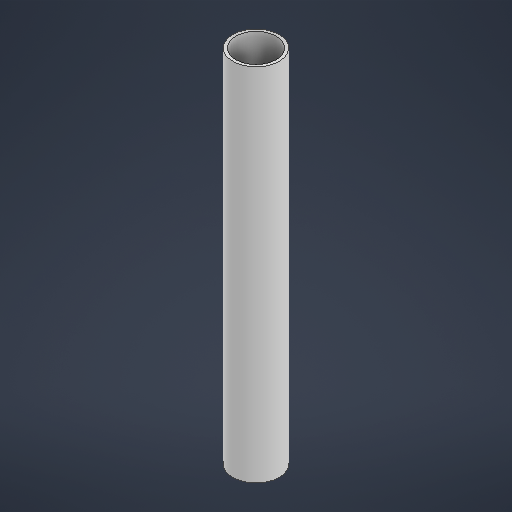
# Autodesk Inventor part: Fuel Tank
Saved by Autodesk Inventor 2026 (Build 300175050, 175E)
## iProperties
Created: 2026-03-18
Part Number: Fuel Tank
Material: Generic
Document SubType Name: Modeling
Designer: jackr
Density: 1 g/cm^3
Appearance: Default
Tank_Outer_Diameter_NO: 12.000 in
Tank_Inner_Diameter_NO: 10.510 in
Tank_Outer_Diameter: 12.000 in
Tank_Inner_Diameter: 10.514 in
Tank_Shell_Height: 93.169 in
Outlet_Cap_Knuckle_Radius: 1.852 in
Outlet_Cap_Crown_Radius: 9.803 in
Outlet_Cap_Skirt_Length: 0.500 in
Author: jackr
Autodesk Inventor part; units mm, degrees
ref_plane "YZ Plane" through (0, 0, 0) normal (1, 0, 0) x (0, 1, 0)
ref_plane "XZ Plane" through (0, 0, 0) normal (0, 1, 0) x (-1, 0, 0)
ref_plane "XY Plane" through (0, 0, 0) normal (0, 0, 1) x (1, 0, 0)
sketch "Sketch1" plane through (0, 0, 0) normal (0, 1, 0) x (-1, 0, 0)
  circle A0 centre (0, 0) radius 133.477
  circle A1 centre (0, 0) radius 152.4
  dimension "Tank_Outer_Diameter_NO" = 304.8
  dimension "Tank_Inner_Diameter_NO" = 266.954
  constraints: 2 centre point, 2 coincident
  measures "Tank_Outer_Diameter_NO" diameter of A1
  measures "Tank_Inner_Diameter_NO" diameter of A0
extrude "Extrusion1" add sketch "Sketch1" along normal blind 2366.4863
equation "\"Tank_Shell_Height_NO\" = Tank_Shell_Height"
equation "\"Outlet_Cap_Wall_Thickness\" = 14.06223"
equation "\"Tank_Outer_Diameter\" = 304.8"
equation "\"Tank_Inner_Diameter\" = 267.06128"
equation "\"Tank_Shell_Height\" = 2366.48629"
equation "\"Outlet_Cap_Knuckle_Radius\" = 47.03484"
equation "\"Outlet_Cap_Crown_Radius\" = 249.00798"
equation "\"Outlet_Cap_Skirt_Length\" = 12.7"
body "Solid1"
